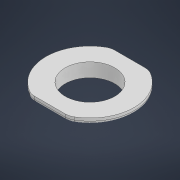
# Autodesk Inventor part: FilterPort_Printable
Saved by Autodesk Inventor 2021 (Build 250183000, 183)
## iProperties
Created: 2020-05-23
Part Number: FilterPort_Printable
Material: Generic
Document SubType Name: Modeling
Designer: Shadow
Density: 1 g/cm^3
Appearance: Default
Author: Shadow
Autodesk Inventor part; units mm, degrees
ref_plane "YZ Plane" through (0, 0, 0) normal (1, 0, 0) x (0, 1, 0)
ref_plane "XZ Plane" through (0, 0, 0) normal (0, 1, 0) x (-1, 0, 0)
ref_plane "XY Plane" through (0, 0, 0) normal (0, 0, 1) x (1, 0, 0)
sketch "Sketch1" plane through (0, 0, 0) normal (0, 1, 0) x (-1, 0, 0)
  circle A0 centre (0, 0) radius 10 construction
  circle A1 centre (0, 0) radius 16
  circle A2 centre (0, 0) radius 11
  circle A3 centre (0, 0) radius 9
  dimension "d0" = 20
  dimension "d1" = 6
  dimension "d4" = 1
  dimension "d9" = 2
  constraints: 4 centre point, 1 coincident
  measures "d0" diameter of A0
  measures "d1" radial gap between concentric circles of A0 A1
  measures "d4" radial gap between concentric circles of A0 A2
  measures "d9" radial gap between concentric circles of A2 A3
extrude "Extrusion1" add sketch "Sketch1" along normal blind 2 contours A1 | A2 | A3
extrude "Extrusion2" add sketch "Sketch1" against normal blind 3 contours A2 | A3
extrude "Extrusion4" cut sketch "Sketch1" along normal through all both and the other way through all contours A3
sketch "Sketch4" plane through (0, 2, 0) normal (0, 1, 0) x (1, 0, 0)
  circle A0 centre (0, 0) radius 16 projected
  line L0 (16, -14.5) -> (-16, -14.5)
  line L1 (-16, -14.5) -> (-16, 14.5)
  line L2 (-16, 14.5) -> (16, 14.5)
  line L3 (16, 14.5) -> (16, -14.5)
  line L4 (16, -14.5) -> (-16, 14.5) construction
  line L5 (-16, -14.5) -> (16, 14.5) construction
  line L6 (-17.5, -16) -> (17.5, -16)
  line L7 (17.5, -16) -> (17.5, 16)
  line L8 (17.5, 16) -> (-17.5, 16)
  line L9 (-17.5, 16) -> (-17.5, -16)
  dimension "d18" = 29
  constraints: 20 end point, 4 parallel, 2 midpoint, 2 perpendicular, 2 tangent, 1 horizontal, 3 other
  measures "d18" distance of L0.end L1.end
extrude "Extrusion6" cut sketch "Sketch4" against normal up to surface (2 mm away) contours L3 L2 A0 L8 L7 L6 L0 | L2 A0 | A0 L0 | A0 L2 L1 L0 L6 L9 L8
fillet "Fillet1" radius 5 4 edges at (-6.7639, 1, 14.5) (6.7639, 1, 14.5) (-6.7639, 1, -14.5) (6.7639, 1, -14.5)
fillet "Fillet2" radius 1 8 edges at (-6.8509, 0, 14.3265) (6.8509, 0, 14.3265) (0, 0, 14.5) (-16, 0, 0) (16, 0, 0) (-6.8509, 0, -14.3265) (6.8509, 0, -14.3265) (0, 0, -14.5)
equation "\"d0\" = FilterDia"
equation "\"MaskHeight\" = 125"
equation "\"FilterDia\" = 20"
equation "\"NoseWidth\" = 25"
equation "\"MaterialThickness\" = 2"
equation "\"Tol\" = 0.25"
equation "\"MaterialHardness\" = 0.3"
equation "\"ClipHeight\" = 4"
equation "\"ClipWidth\" = 5"
equation "\"ClipNeck\" = 5"
equation "\"ValveNeckDia\" = 3"
equation "\"ValveNeckLength\" = 2"
equation "\"ValveFlapDia\" = 19.25"
equation "\"LeftValve\" = 0"
equation "\"RightValve\" = 0"
equation "\"CoreScrewHeadDia\" = 9.525"
equation "\"CoreScrewLength\" = 50.8"
equation "\"CoreScrewID\" = 2.38125"
equation "\"CoreScrewOD\" = 3.96875"
equation "\"StrapAttachmentNeckDia\" = 6.5"
equation "\"StrapAttachmentNeckHeight\" = 1.5"
equation "\"StrapNoseRadialDifference\" = 2"
equation "\"StrapNoseHeight\" = 7.5"
equation "\"ZipTieThickness\" = 4"
equation "\"PinTol\" = 0.75"
equation "\"PinDia\" = 7"
equation "\"PinDepth\" = 5"
body "Solid1"
